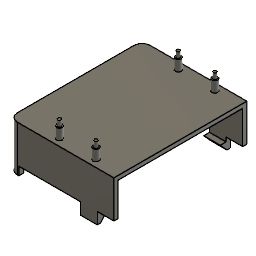
3rdfloor (Autodesk Fusion 360 design; units mm, degrees)
Autodesk Fusion 360 part; units mm, degrees
sketch "Sketch1" plane through (0, 0, 0) normal (0, 1, 0) x (1, 0, 0)
  line L0 (54.5, 40) -> (-54.5, 40)
  line L1 (-54.5, 40) -> (-54.5, -40)
  line L2 (-54.5, -40) -> (54.5, -40)
  line L3 (54.5, -40) -> (54.5, 40)
  line L4 (54.5, 40) -> (-54.5, -40) construction
  line L5 (-54.5, 40) -> (54.5, -40) construction
  line L6 (53.5, 37.5) -> (-46, 37.5)
  line L7 (-53.5, 30) -> (-53.5, -30)
  line L8 (-46, -37.5) -> (53.5, -37.5)
  line L9 (53.5, -37.5) -> (53.5, 37.5)
  line L10 (53.5, 37.5) -> (-53.5, -37.5) construction
  line L11 (-53.5, 37.5) -> (53.5, -37.5) construction
  line L12 (8.5, 52.9036) -> (8.5, -63.6851)
  arc A0 (-53.5, -30) -> (-46, -37.5) centre (-46, -30) ccw
  arc A1 (-46, 37.5) -> (-53.5, 30) centre (-46, 30) ccw
  line L13 (-48.6203, 43.8236) -> (-48.6203, -44.4257)
  line L14 (-1.5, -37.5) -> (-1.5, -40)
  line L15 (-11.5, -37.5) -> (-11.5, -40)
  line L16 (-11.5, 40) -> (-11.5, 37.5)
  line L17 (-1.5, 40) -> (-1.5, 37.5)
  dimension "d1" = 109
  dimension "d4" = 107
  dimension "d5" = 75
  dimension "d10" = 45
  dimension "d13" = 7.5
  dimension "d22" = 2.5
  dimension "d23" = 10
  dimension "d24" = 10
  dimension "d25" = 10
  dimension "d26" = 10
  constraint horizontal L0
  constraint perpendicular L0 L1
  constraint parallel L0 L2
  constraint parallel L1 L3
  constraint coincident L4 origin
  constraint coincident L5 origin
  constraint horizontal L6
  constraint perpendicular L6 L7
  constraint parallel L6 L8
  constraint parallel L7 L9
  constraint coincident L10 origin
  constraint coincident L11 origin
  constraint perpendicular L0 L12
  constraint coincident L10.end L8
  constraint coincident L10.end L7
  constraint tangent L8 A0
  constraint tangent L7 A0
  constraint coincident L11.start L7
  constraint coincident L11.start L6
  constraint tangent L7 A1
  constraint tangent L6 A1
  constraint equal A0 A1
  constraint perpendicular L2 L13
  constraint coincident L8 L14.start
  constraint coincident L2 L14.end
  constraint perpendicular L2 L14
  constraint coincident L8 L15.start
  constraint coincident L2 L15.end
  constraint perpendicular L2 L15
  constraint coincident L0 L16.start
  constraint coincident L6 L16.end
  constraint perpendicular L6 L16
  constraint coincident L0 L17.start
  constraint coincident L6 L17.end
  constraint perpendicular L6 L17
  measures "d1" distance of L0.start L0.end
  measures "d4" distance of L10.end L8.end
  measures "d5" distance of L11.start L10.end
  measures "d10" distance of L9 L12
  measures "d13" radius of A0
  measures "d22" distance of L0 L6
  measures "d23" distance of L14 L15
  measures "d24" distance of L12 L14
  measures "d25" distance of L16 L17
  measures "d26" distance of L12 L17
extrude "Extrude1" add sketch "Sketch1" against normal blind 20 contours L0 L6 L16 L17 | L0 L6 L12 L17 | L0 L6 A1 L13 L16 | L0 L1 L2 L7 A0 A1 L13 | L2 L8 L12 L14 | L2 L8 A0 L13 L15 | L2 L8 L14 L15
extrude "Extrude2" add sketch "Sketch1" along normal blind 2.5 contours L0 L6 L16 L17 | L0 L6 L12 L17 | L0 L6 A1 L13 L16 | L6 L8 L12 A0 A1 L13 | L0 L1 L2 L7 A0 A1 L13 | L7 A0 A1 L13 | L2 L8 L12 L14 | L2 L8 A0 L13 L15 | L2 L8 L14 L15
extrude "Extrude3" add sketch "Sketch1" against normal blind 25 contours L0 L1 L2 L7 A0 A1 L13
fillet "Fillet2" radius 5 2 edges at (-54.5, -11.25, -40) (-54.5, -11.25, 40)
sketch "Sketch2" plane through (-54.5, 0, 0) normal (-1, 0, 0) x (0, 0, 1)
  line L0 (35, -25) -> (35, 2.5)
  line L1 (35, 2.5) -> (-35, 2.5)
  line L2 (-35, 2.5) -> (-35, -25)
  line L3 (-35, -25) -> (35, -25)
  line L4 (-30, -25) -> (30, -25)
  line L5 (30, -25) -> (30, -1.1798)
  line L6 (30, -1.1798) -> (-30, -1.1798)
  line L7 (-30, -1.1798) -> (-30, -25)
  dimension "d18" = 60
  dimension "d19" = 30
  constraint horizontal L4
  constraint vertical L5
  constraint horizontal L6
  constraint vertical L7
  constraint coincident L3 L4.start
  measures "d18" distance of L5 L7
  measures "d19" distance of L5 origin
extrude "Extrude4" cut sketch "Sketch2" against normal blind 10 contours L3 L4 L5 L6 L7
extrude "Extrude5" add sketch "Sketch1" against normal blind 22.5 contours L0 L6 L16 L17 | L2 L8 L14 L15
sketch "Sketch3" plane through (-1.5, 0, 0) normal (1, 0, 0) x (0, 0, -1)
  line L0 (-37.5, -20) -> (-40, -20)
  line L1 (-40, -20) -> (-40, -22.5)
  line L2 (-40, -22.5) -> (-37.5, -22.5)
  line L3 (-37.5, -22.5) -> (-37.5, -20)
  line L4 (-37.5, -22.5) -> (-34, -22.5)
  line L5 (-40, -22.5) -> (-40, -27)
  line L6 (-40, -27) -> (-37.9698, -27)
  line L7 (-37.9698, -27) -> (-34, -22.5)
  dimension "d29" = 3.5
  dimension "d30" = 4.5
  constraint coincident L2.end L3.start
  constraint perpendicular L3 L4
  constraint coincident L1.end L2.start
  constraint perpendicular L2 L5
  constraint perpendicular L5 L6
  measures "d29" distance of L2.end L4.end
  measures "d30" distance of L1.end L5.end
extrude "Extrude6" add sketch "Sketch3" against normal blind 10 contours L2 L4 L5 L6 L7
mirror "Mirror1" about plane through (0, 0, 0) normal (0, 0, 1) of "Extrude6"
sketch "Sketch4" plane through (0, 2.5, 0) normal (0, 1, 0) x (-1, 0, 0)
  arc A0 (54.5, 35) -> (49.5, 40) centre (49.5, 35) ccw
  line L0 (49.5, 40) -> (-8.5, 40)
  line L1 (-8.5, 40) -> (-8.5, -40)
  line L2 (-8.5, -40) -> (49.5, -40)
  arc A1 (49.5, -40) -> (54.5, -35) centre (49.5, -35) ccw
  line L3 (54.5, -35) -> (54.5, 35)
  circle A2 centre (6.5, -35.75) radius 1
  circle A3 centre (6.5, -35.75) radius 1.75
  circle A4 centre (28.5, -35.75) radius 1
  circle A5 centre (28.5, -35.75) radius 1.75
  circle A6 centre (6.5, 35.75) radius 1
  circle A7 centre (6.5, 35.75) radius 1.75
  circle A8 centre (28.5, 35.75) radius 1
  circle A9 centre (28.5, 35.75) radius 1.75
  dimension "d35" = 2
  dimension "d36" = 3.5
  dimension "d39" = 22
  dimension "d40" = 71.5
  dimension "d41" = 4.25
  dimension "d42" = 4.25
  dimension "d43" = 15
  constraint concentric A2 A3
  measures "d35" diameter of A2
  measures "d36" diameter of A3
  measures "d41" distance of L2 A4.centre
  measures "d42" distance of L0 A8.centre
  measures "d43" distance of L1 A2.centre
extrude "Extrude7" add sketch "Sketch4" along normal blind 6.5 contours A2 | A3 | A4 | A5 | A6 | A7 | A8 | A9
extrude "Extrude8" add sketch "Sketch4" along normal blind 10 contours A2 | A4 | A6 | A8
equation "d19 = d18 / 2"
equation "d25 = d23"
equation "d26 = d24"
equation "d41 = d42"
equation "d46 = 6.5 mm + 3.5 mm"
